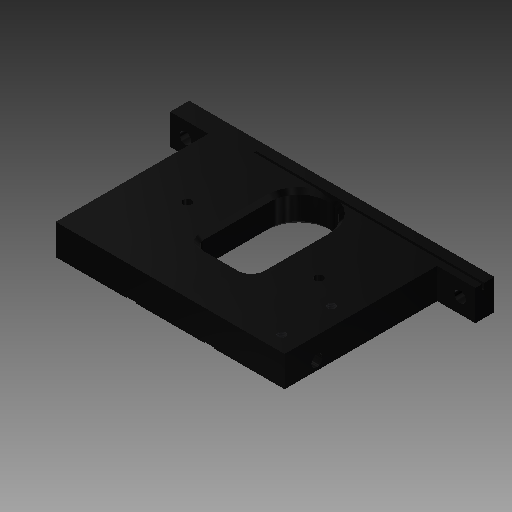
# Autodesk Inventor part: Türwand2
Saved by Autodesk Inventor 2018 (Build 220112000, 112)
## iProperties
Created: 2012-12-05
Part Number: Türwand2
Material: Polycarbonate, Clear
Document SubType Name: Modeling
Designer: Neef
Density: 1.2 g/cm^3
Mass: 185.178 g
Surface Area: 361.082 cm^2
Volume: 154.315 cm^3
Appearance: Glossy - Black
Author: Neef
Autodesk Inventor part; units mm, degrees
ref_plane "YZ Plane" through (0, 0, 0) normal (1, 0, 0) x (0, 1, 0)
ref_plane "XZ Plane" through (0, 0, 0) normal (0, 1, 0) x (-1, 0, 0)
ref_plane "XY Plane" through (0, 0, 0) normal (0, 0, 1) x (1, 0, 0)
sketch "Skizze1" plane through (0, 0, 0) normal (0, 0, 1) x (1, 0, 0)
  line L0 (-60, -45) -> (60, -45)
  line L1 (60, -45) -> (60, 45)
  line L2 (60, 45) -> (-60, 45)
  line L3 (-60, 45) -> (-60, -45)
  line L4 (0, 63) -> (0, -63) projected
  line L5 (-84, 0) -> (84, 0) projected
  point P0 (0, 0)
  point P1 (-60, 0)
  point P2 (0, -45)
  dimension "d0" = 90
  dimension "d1" = 120
  constraints: 8 end point, 2 midpoint, 2 parallel, 2 point on line, 1 horizontal, 1 perpendicular
  measures "d0" distance of L2.end L0.start
  measures "d1" distance of L1.end L2.end
extrude "Extrusion1" add sketch "Skizze1" along normal blind 30
sketch "Skizze2" plane through (0, 0, 30) normal (0, 0, 1) x (1, 0, 0)
  line L0 (-60, -45) -> (-60, 45) projected
  line L1 (60, 45) -> (60, -45) projected
  line L2 (-60, 39.7) -> (60, 39.7)
  line L3 (-60, 38.5) -> (60, 38.5)
  line L4 (-60, 45) -> (60, 45) projected
  point P0 (0, 0)
  dimension "d4" = 1.2
  dimension "d17" = 6.5
  constraints: 4 end point, 4 point on line, 2 perpendicular
  measures "d4" distance between parallel lines of L2 L3
  measures "d17" distance between parallel lines of L4 L3
extrude "Extrusion2" cut sketch "Skizze2" against normal blind 3 contours L0 L2 L1 L3
sketch "Skizze3" plane through (0, 0, 30) normal (0, 0, 1) x (1, 0, 0)
  line L0 (15, 22.5) -> (15, -12.5)
  line L1 (10, -17.5) -> (-10, -17.5)
  line L2 (-15, -12.5) -> (-15, 22.5)
  arc A0 (-15, -12.5) -> (-10, -17.5) centre (-10, -12.5) ccw
  arc A1 (10, -17.5) -> (15, -12.5) centre (10, -12.5) ccw
  line L3 (60, 38.5) -> (-60, 38.5) projected
  line L4 (60, 45) -> (60, 39.7) projected
  arc A2 (15, 22.5) -> (-15, 22.5) centre (0, 22.5) ccw
  point P0 (0, 0)
  point P1 (-15, 37.5)
  point P2 (15, 37.5)
  point P3 (-15, -17.5)
  point P4 (0, 37.5)
  dimension "d8" = 30
  dimension "d9" = 55
  dimension "d10" = 15
  dimension "d18" = 5
  dimension "d19" = 15
  dimension "d20" = 90
  dimension "d21" = 90
  dimension "d22" = 62.5
  dimension "d23" = 16
  dimension "d24" = 60
  constraints: 7 point on circle, 6 end point, 6 tangent, 4 point on line, 3 centre point, 1 equal radius, 1 parallel
  measures "d8" distance of point (-15, 37.5) point (15, 37.5)
  measures "d9" distance of point (-15, -17.5) point (-15, 37.5)
  measures "d10" distance from line of L2 point (0, 0)
  measures "d18" radius of A1
  measures "d19" radius of A2
  measures "d20" angle of L4 L1
  measures "d21" angle of L3 L2
  measures "d22" distance from line of L4.start L1
  measures "d23" distance from line of L0.start L3
  measures "d24" distance from line of point (0, 37.5) L4
extrude "Extrusion3" cut sketch "Skizze3" against normal up to surface (30 mm away)
chamfer "Fase1" distance 2 angle 45 6 edges at (0, 37.5, 30) (15, 5, 30) (13.5355, -16.0355, 30) (0, -17.5, 30) (-13.5355, -16.0355, 30) (-15, 5, 30)
sketch "Skizze5" plane through (0, 0, 0) normal (0, 0, -1) x (-1, 0, 0)
  arc A0 (15, 22.5) -> (-15, 22.5) centre (0, 22.5) ccw projected
  line L0 (10, -17.5) -> (-10, -17.5) projected
  line L1 (-15, -12.5) -> (-15, 22.5) projected
  line L2 (60, -45) -> (-60, -45) projected
  line L3 (0, -35.5) -> (-11, -35.5)
  line L4 (-11, -35.5) -> (-11, -20.5)
  line L5 (-11, -20.5) -> (0, -20.5)
  line L6 (0, -20.5) -> (0, -35.5)
  line L7 (0, 22.5) -> (0, -45) construction
  point P0 (0, 0)
  dimension "d28" = 4
  dimension "d29" = 3
  dimension "d30" = 15
  constraints: 10 end point, 2 parallel, 2 perpendicular, 1 collinear, 1 midpoint
  measures "d28" distance between parallel lines of L4 L1
  measures "d29" distance between parallel lines of L5 L0
  measures "d30" distance of L3.end L4.end
extrude "Extrusion4" cut sketch "Skizze5" against normal blind 25
sketch "Skizze6" plane through (0, 0, 0) normal (0, 0, -1) x (-1, 0, 0)
  line L0 (0, -20.5) -> (0, -35.5) projected
  line L1 (0, -35.5) -> (-11, -35.5) projected
  line L2 (-11, -35.5) -> (-11, -20.5) projected
  line L3 (-11, -20.5) -> (0, -20.5) projected
  arc A0 (15, 22.5) -> (-15, 22.5) centre (0, 22.5) ccw projected
  line L4 (10, -17.5) -> (-10, -17.5) projected
  arc A1 (-15, -12.5) -> (-10, -17.5) centre (-10, -12.5) ccw projected
  line L5 (-15, -12.5) -> (-15, 22.5) projected
  line L6 (-60, 45) -> (60, 45) projected
  line L7 (-60, -45) -> (-60, 45) projected
  line L8 (60, -45) -> (-60, -45) projected
  line L9 (0, 45) -> (0, -45) construction
  line L10 (-18, -45) -> (-18, 22.5)
  arc A2 (0, 40.5) -> (-18, 22.5) centre (0, 22.5) ccw
  line L11 (-23, -45) -> (-23, 22.5)
  arc A3 (-4.7697, 45) -> (-23, 22.5) centre (0, 22.5) ccw
  line L12 (0, -17.5) -> (0, -45)
  line L13 (0, -35.5) -> (-11, -35.5)
  line L14 (-11, -20.5) -> (0, -20.5)
  line L15 (-11, -20.5) -> (-11, -35.5)
  line L16 (-23, -45) -> (-18, -45)
  line L17 (-4.7697, 45) -> (0, 45)
  line L18 (0, 45) -> (0, 40.5)
  line L19 (0, 40.5) -> (0, 37.5)
  point P0 (0, 0)
  dimension "d33" = 3
  dimension "d34" = 18
  dimension "d35" = 23
  dimension "d36" = 5
  dimension "d37" = 67.5
  constraints: 22 end point, 7 point on line, 5 collinear, 5 point on circle, 3 midpoint, 3 parallel, 2 centre point, 2 perpendicular, 1 tangent
  measures "d33" distance between parallel lines of L5 L10
  measures "d34" radius of A2
  measures "d35" radius of A3
  measures "d36" distance between parallel lines of L10 L11
  measures "d37" distance of L10.start L10.end
extrude "Extrusion5" cut sketch "Skizze6" against normal blind 14 contours L3 L2 L1 L12 L8 L10 A2 L19 A0 L5 A1 L4 | L8 L7 L6 A3 L11
mirror "Spiegeln1" about plane through (0, -35.5, 0) normal (1, 0, 0) of "Extrusion5", "Extrusion4"
chamfer "Fase2" distance 2 angle 45 6 edges at (0, -17.5, 14) (-13.5355, -16.0355, 14) (-15, 5, 14) (0, 37.5, 14) (15, 5, 14) (13.5355, -16.0355, 14)
sketch "Skizze7" plane through (0, 0, 14) normal (0, 0, -1) x (-1, 0, 0)
  line L0 (-11, -20.5) -> (-11, -35.5) projected
  line L1 (11, -20.5) -> (-11, -20.5)
  line L2 (-11, -20.5) -> (-11, -16.6845)
  line L3 (-11, -16.6845) -> (11, -16.6845)
  line L4 (11, -16.6845) -> (11, -20.5)
  point P0 (0, 0)
  constraints: 8 end point, 2 parallel, 1 horizontal, 1 perpendicular, 1 point on line
extrude "Extrusion6" cut sketch "Skizze7" against normal blind 5
fillet "Rundung1" radius 2 4 edges at (-11, -20.5, 22) (-11, -35.5, 19.5) (11, -35.5, 19.5) (11, -20.5, 22)
sketch "Skizze8" plane through (60, -45, 30) normal (1, 0, 0) x (0, 0, -1)
  line L0 (16, 9.5) -> (5, 9.5) projected
  line L1 (5, 24.5) -> (11, 24.5) projected
  line L2 (14, 27.601) -> (11, 27.601) projected
  line L3 (16, 25.5718) -> (16, 11.5) projected
  line L4 (5, 22.5) -> (5, 11.5) projected
  line L5 (5, 9.5) -> (5, 11.5) projected
  line L6 (11, 27.601) -> (11, 27.5) projected
  line L7 (2, 27.5) -> (11, 27.5) projected
  line L8 (2, 32.5) -> (2, 27.5) projected
  line L9 (2, 32.5) -> (14, 32.5) projected
  line L10 (14, 27.601) -> (14, 32.5) projected
  line L11 (14, 27.601) -> (11, 27.601) projected
  circle A0 centre (11.5, 17) radius 2.25 construction
  circle A1 centre (11.5, 17) radius 4 construction
  line L12 (11, 27.601) -> (11, 27.5) construction
  line L13 (11, 22.5) -> (11, 27.601) construction
  line L14 (11, 24.5) -> (11, 22.5) construction
  line L15 (11, 22.5) -> (11, 24.5) construction
  line L16 (11, 27.601) -> (11, 22.5) construction
  line L17 (11, 27.5) -> (11, 27.601) construction
  line L18 (16, 25.5718) -> (16, 11.5) construction
  line L19 (16, 32.5) -> (16, 25.5718) construction
  line L20 (16, 67.5) -> (16, 32.5) construction
  line L21 (16, 67.5) -> (16, 67.5) construction
  line L22 (16, 32.5) -> (16, 67.5) construction
  line L23 (16, 25.5718) -> (16, 32.5) construction
  line L24 (16, 25.5718) -> (16, 11.5) construction
  line L25 (16, 9.5) -> (16, 11.5) construction
  line L26 (16, 11.5) -> (16, 9.5) construction
  line L27 (16, 67.5) -> (16, 67.5) construction
  line L28 (16, 67.5) -> (16, 0) construction
  line L29 (16, 67.5) -> (16, 0) construction
  point P0 (30, 45)
  dimension "d46" = 4.5
  dimension "d47" = 8
  dimension "d48" = 6.5
  dimension "d49" = 7.5
  constraints: 2 centre point, 2 coincident, 1 other
  measures "d46" diameter of A0
  measures "d47" diameter of A1
  measures "d48" distance from line of L4 point (11.5, 17)
  measures "d49" distance from line of L0 point (11.5, 17)
hole "Bohrung1" at (60, -28, 18.5) direction (-1, 0, 0) diameter 6 end through all
sketch "Skizze9" plane through (-60, 45, 30) normal (0, 1, 0) x (1, 0, 0)
  line L0 (0, 16) -> (-20, 16)
  line L1 (-20, 16) -> (-20, 0)
  line L2 (-20, 0) -> (0, 0)
  line L3 (0, 0) -> (0, 16)
  point P0 (60, 30)
  dimension "d57" = 20
  dimension "d58" = 16
  constraints: 8 end point, 2 parallel, 1 horizontal, 1 perpendicular
  measures "d57" distance of L0.start L0.end
  measures "d58" distance of L0.end L1.end
extrude "Extrusion7" add sketch "Skizze9" against normal blind 10
sketch "Skizze10" plane through (-60, 35, 30) normal (0, -1, 0) x (1, 0, 0)
  line L0 (-20, -16) -> (-20, 0) projected
  point P0 (60, -30)
  point P1 (-12, -8)
  dimension "d61" = 8
  measures "d61" distance from line of L0 point (-12, -8)
hole "Bohrung2" at (-72, 35, 22) direction (0, 1, 0) diameter 6 end through all
mirror "Spiegeln2" about plane through (0, 0, 0) normal (1, 0, 0) of "Extrusion7", "Bohrung2"
move faces "Fläche verschieben1" translate (20, 0, 0) faces at (60, 39.3, 29)
move faces "Fläche verschieben2" translate (20.5, 0, 0) faces at (-60, 39.3, 29)
sketch "Skizze11" plane through (0, 0, 14) normal (0, 0, -1) x (-1, 0, 0)
  line L0 (-23, -45) -> (-23, 22.5) projected
  line L1 (-80, 45) -> (-4.7697, 45) projected
  circle A0 centre (-34.5, -1.5) radius 1.621 projected
  point P0 (0, 0)
  point P1 (-34.5, -1.5)
  dimension "d69" = 11.5
  dimension "d70" = 46.5
  measures "d69" distance from line of L0 point (-34.5, -1.5)
  measures "d70" distance from line of L1 point (-34.5, -1.5)
hole "Bohrung3" at (34.5, -1.5, 14) direction (0, 0, 1) diameter 4.4 end through all
mirror "Spiegeln3" about plane through (0, 0, 0) normal (1, 0, 0) of "Bohrung3"
sketch "Skizze12" plane through (0, 0, 30) normal (0, 0, 1) x (1, 0, 0)
  line L0 (60, -45) -> (-60, -45) projected
  line L1 (60, 35) -> (60, -45) projected
  point P0 (0, 0)
  point P1 (50.5, -37)
  point P2 (50.5, -11)
  dimension "d78" = 9.5
  dimension "d79" = 9.5
  dimension "d80" = 8
  dimension "d81" = 34
  measures "d78" distance from line of L1 point (50.5, -37)
  measures "d79" distance from line of L1 point (50.5, -11)
  measures "d80" distance from line of L0 point (50.5, -37)
  measures "d81" distance from line of L0 point (50.5, -11)
hole "Bohrung4" at (50.5, -37, 30) at (50.5, -11, 30) direction (0, 0, -1) diameter 4.134 end through all thread size "M5x0.8" class "6H" standard "ISO Metric profile"
move faces "Fläche verschieben3" translate (0, 0, 14.5) faces at (-19.6667, 0, 0)
sketch "Skizze13" plane through (4.7697, 45, 14.5) normal (0, 0, -1) x (-1, 0, 0)
  line L0 (22.7697, -22.5) -> (22.7697, -90) projected
  line L1 (27.7697, -90) -> (22.7697, -90) projected
  line L2 (-13.2303, -90) -> (-13.2303, -22.5) projected
  line L3 (-18.2303, -90) -> (-55.2303, -90) projected
  point P0 (4.7697, -45)
  point P1 (-15.7303, -50)
  point P2 (25.2697, -50)
  dimension "d89" = 40
  dimension "d90" = 40
  dimension "d91" = 2.5
  dimension "d92" = 2.5
  measures "d89" distance from line of L3 point (-15.73, -50)
  measures "d90" distance from line of L1 point (25.27, -50)
  measures "d91" distance from line of L2 point (-15.73, -50)
  measures "d92" distance from line of point (25.27, -50) L0
hole "Bohrung5" at (20.5, -5, 14.5) at (-20.5, -5, 14.5) direction (0, 0, 1) diameter 2.459 depth 10 tip angle 118 thread size "M3x0.5" class "6H" standard "ISO Metric profile"
equation "\"d10\" = 0.5 * d8"
equation "\"d79\" = d78"
equation "\"d90\" = d89"
equation "\"d92\" = d91"
